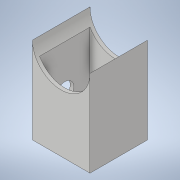
# Autodesk Inventor part: Seat tab to frame mount
Saved by Autodesk Inventor 2021 (Build 250183000, 183)
## iProperties
Created: 2019-10-29
Part Number: Seat tab to frame mount
Material: Generic
Description: Cockpit tab
Document SubType Name: Modeling
Designer: fagang
Density: 1 g/cm^3
Appearance: Default
Material_Size: 1/16" thick square steel tubing
Quantity: 4
Author: fagang
Autodesk Inventor part; units mm, degrees
ref_plane "YZ Plane" through (0, 0, 0) normal (1, 0, 0) x (0, 1, 0)
ref_plane "XZ Plane" through (0, 0, 0) normal (0, 1, 0) x (-1, 0, 0)
ref_plane "XY Plane" through (0, 0, 0) normal (0, 0, 1) x (1, 0, 0)
sketch "Sketch3" plane through (0, 0, 0) normal (0, 1, 0) x (-1, 0, 0)
  line L0 (2.7739, 2.9) -> (-22.6261, 2.9)
  line L1 (-22.6261, 2.9) -> (-22.6261, -22.5)
  line L2 (-22.6261, -22.5) -> (2.7739, -22.5)
  line L3 (2.7739, -22.5) -> (2.7739, 2.9)
  line L4 (-22.6261, 2.9) -> (-21.0386, 2.9)
  line L5 (-21.0386, -20.9125) -> (1.1864, -20.9125)
  line L6 (1.1864, -20.9125) -> (1.1864, 1.3125)
  line L7 (1.1864, 1.3125) -> (-21.0386, 1.3125)
  line L8 (-21.0386, 1.3125) -> (-21.0386, -20.9125)
  point P0 (0, 0)
  dimension "d4" = 25.4
  dimension "d5" = 25.4
  dimension "d6" = 1.5875
  dimension "d7" = 23.8125
  dimension "d8" = 22.225
  dimension "d9" = 22.225
  constraints: 18 end point, 3 parallel, 2 perpendicular, 1 horizontal, 1 point on line, 1 vertical
  measures "d4" distance of L2.end L1.end
  measures "d5" distance of L1.end L0.end
  measures "d6" distance of L0.end L4.end
  measures "d7" distance of L4.end L5.start
  measures "d8" distance of L5.start L5.end
  measures "d9" distance of L5.end L6.end
extrude "Extrusion2" add sketch "Sketch3" along normal blind 38.1
sketch "Sketch5" plane through (-2.7739, 0, 2.9) normal (0, 0, 1) x (1, 0, 0)
  line L0 (0, 38.1) -> (25.4, 38.1) projected
  circle A0 centre (12.7, 38.1) radius 12.7
  point P0 (2.7739, 0)
  constraints: 1 horizontal alignment, 1 midpoint, 2 other
extrude "Extrusion4" cut sketch "Sketch5" against normal blind 25.4
sketch "Sketch8" plane through (-2.7739, 0, -22.5) normal (-1, 0, 0) x (0, 0, 1)
  circle A0 centre (12.7, 12.7079) radius 3.9751
  point P0 (22.5, 0)
  dimension "d22" = 7.9502
  constraints: 1 centre point
  measures "d22" diameter of A0
extrude "Extrusion6" cut sketch "Sketch8" against normal blind 12.7
body "Solid2"
